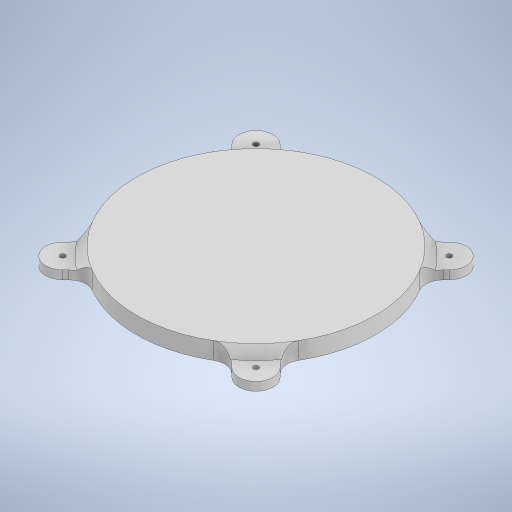
# Autodesk Inventor part: BasePlate
Saved by Autodesk Inventor 2023 (Build 270158030, 158C)
## iProperties
Created: 2024-09-25
Part Number: BasePlate
Material: Generic
Document SubType Name: Modeling
Designer: lvrectanus0
Density: 1 g/cm^3
Appearance: Default
Author: lvrectanus0
Autodesk Inventor part; units mm, degrees
ref_plane "YZ Plane" through (0, 0, 0) normal (1, 0, 0) x (0, 1, 0)
ref_plane "XZ Plane" through (0, 0, 0) normal (0, 1, 0) x (-1, 0, 0)
ref_plane "XY Plane" through (0, 0, 0) normal (0, 0, 1) x (1, 0, 0)
sketch "Sketch1" plane through (0, 0, 0) normal (0, 1, 0) x (-1, 0, 0)
  circle A0 centre (0, 0) radius 88.9
  dimension "d0" = 177.8
  constraints: 1 centre point, 1 coincident
  measures "d0" diameter of A0
extrude "Extrusion1" add sketch "Sketch1" along normal blind 6.35
sketch "Sketch2" plane through (0, 0, 0) normal (0, -1, 0) x (1, 0, 0)
  line L0 (-71.842, 71.842) -> (71.842, -71.842) construction
  line L1 (-80.8223, 62.8618) -> (62.8618, -80.8223)
  line L2 (80.8223, -62.8618) -> (-62.8618, 80.8223)
  arc A0 (-62.8618, 80.8223) -> (-80.8223, 62.8618) centre (-71.842, 71.842) ccw
  arc A1 (62.8618, -80.8223) -> (80.8223, -62.8618) centre (71.842, -71.842) ccw
  line L3 (0, 0) -> (203.2, 0) construction
  circle A2 centre (0, 0) radius 88.9 projected
  line L4 (-71.842, -71.842) -> (71.842, 71.842) construction
  line L5 (-62.8618, -80.8223) -> (80.8223, 62.8618)
  line L6 (62.8618, 80.8223) -> (-80.8223, -62.8618)
  arc A3 (-80.8223, -62.8618) -> (-62.8618, -80.8223) centre (-71.842, -71.842) ccw
  arc A4 (80.8223, 62.8618) -> (62.8618, 80.8223) centre (71.842, 71.842) ccw
  line L7 (0, 0) -> (203.2, 0) construction
  circle A5 centre (0, 0) radius 88.9 projected
  circle A6 centre (0, 0) radius 88.9
  point P0 (-53.2368, -71.1973)
  point P1 (53.2368, -71.1973)
  point P2 (71.1973, -53.2368)
  point P3 (71.1973, 53.2368)
  point P4 (53.2368, 71.1973)
  point P5 (-53.2368, 71.1973)
  point P6 (-71.1973, 53.2368)
  point P7 (-71.1973, -53.2368)
  dimension "d3" = 45
  dimension "d4" = 25.4
  dimension "d5" = 45
  dimension "d6" = 25.4
  constraints: 20 end point, 10 tangent, 8 point on circle, 5 centre point, 2 equal length, 2 horizontal, 2 midpoint, 2 parallel, 1 coincident
  measures "d3" angle of L0 L3
  measures "d4" diameter of A1
  measures "d5" angle of L7 L4
  measures "d6" diameter of A4
sketch "Sketch3" plane through (0, 0, 0) normal (0, -1, 0) x (1, 0, 0)
  point P0 (0, 0)
extrude "Extrusion2" add sketch "Sketch2" along normal blind 6.35
fillet "Fillet1" radius 12.7 8 edges at (71.1973, -3.175, 53.2368) (71.1973, -3.175, -53.2368) (53.2368, -3.175, 71.1973) (-53.2368, -3.175, 71.1973) (-71.1973, -3.175, -53.2368) (-71.1973, -3.175, 53.2368) (-53.2368, -3.175, -71.1973) (53.2368, -3.175, -71.1973)
chamfer "Chamfer1" distance 6.35 angle 45 12 edges at (-49.2671, 0, -73.9997) (-62.8618, 0, -62.8618) (-73.9997, 0, -49.2671) (-73.9997, 0, 49.2671) (-62.8618, 0, 62.8618) (-49.2671, 0, 73.9997) (49.2671, 0, 73.9997) (62.8618, 0, 62.8618) (73.9997, 0, 49.2671) (73.9997, 0, -49.2671) (62.8618, 0, -62.8618) (49.2671, 0, -73.9997)
sketch "Sketch4" plane through (0, 0, 0) normal (0, 1, 0) x (1, 0, 0)
  arc A0 (-62.8618, 80.8223) -> (-80.8223, 62.8618) centre (-71.842, 71.842) ccw projected
  arc A1 (80.8223, 62.8618) -> (62.8618, 80.8223) centre (71.842, 71.842) ccw projected
  arc A2 (62.8618, -80.8223) -> (80.8223, -62.8618) centre (71.842, -71.842) ccw projected
  arc A3 (-80.8223, -62.8618) -> (-62.8618, -80.8223) centre (-71.842, -71.842) ccw projected
  point P0 (0, 0)
hole "Hole1" at (-71.842, 0, -71.842) at (71.842, 0, -71.842) at (71.842, 0, 71.842) at (-71.842, 0, 71.842) direction (0, -1, 0) diameter 4 end through all
body "Solid1"
